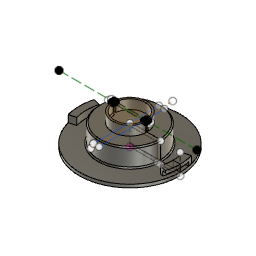
Lantern Disc (Autodesk Fusion 360 design; units mm, degrees)
Autodesk Fusion 360 part; units mm, degrees
note: some values were not read from the file. Set by a fixed rule: which sketch regions a step uses.
sketch "Profile" plane through (0, 0, 0) normal (0, 1, 0) x (1, 0, 0)
  line L0 (16.5, 0) -> (16.5, -11) construction
  line L1 (0, 0) -> (0, -11) construction
  line L2 (27, 0) -> (27, -11) construction
  line L3 (0, 0) -> (27, 0)
  line L4 (27, 0) -> (27, -1.7)
  line L5 (27, -1.7) -> (0, -1.7)
  line L6 (0, -1.7) -> (16.5, -1.7) construction
  line L7 (16.5, -1.7) -> (16.5, -11.5)
  line L8 (16.5, -11.5) -> (0, -11.5)
  line L9 (14.75, 0) -> (14.75, -9.75)
  line L10 (14.75, -9.75) -> (0, -9.75)
  line L11 (0, -11.5) -> (0, -9.75) construction
  line L12 (0, -11.5) -> (0, -9.75)
  line L13 (8.25, -16.5) -> (9.25, -16.5)
  line L14 (9.25, -16.5) -> (9.25, -11.5)
  line L15 (9.25, -11.5) -> (8.25, -11.5)
  line L16 (8.25, -11.5) -> (8.25, -16.5)
  line L17 (25, -3.7) -> (27, -3.7)
  line L18 (25, -3.7) -> (25, -1.7)
  line L19 (23.25, -5.45) -> (23.25, -1.7)
  line L20 (23.25, -5.45) -> (27, -5.45)
  line L21 (27, -5.45) -> (27, -3.7)
  line L22 (27, -3.7) -> (27, -1.7)
  dimension "d29" = 16.5
  dimension "d30" = 27
  dimension "d33" = 1.75
  dimension "d35" = 1.75
  dimension "d36" = 9.25
  dimension "d37" = 1
  dimension "d38" = 2
  dimension "d39" = 1.75
  dimension "d40" = 1.75
  dimension "d41" = 2
  dimension "d42" = 5
  dimension "d55" = 11.5
  dimension "d56" = 1.7
  constraint coincident L1.start L3.start
  constraint horizontal L3
  constraint vertical L4
  constraint horizontal L5
  constraint coincident L2 L4.end
  constraint horizontal L6
  constraint vertical L7
  constraint horizontal L8
  constraint coincident L0 L7.end
  constraint perpendicular L8 L9
  constraint coincident L1 L10.end
  constraint parallel L8 L10
  constraint perpendicular L10 L11
  constraint horizontal L13
  constraint vertical L14
  constraint horizontal L15
  constraint vertical L16
  constraint coincident L8 L14.end
  constraint coincident L2 L17.end
  constraint perpendicular L2 L17
  constraint coincident L5 L18.end
  constraint perpendicular L5 L18
  constraint coincident L5 L19.end
  constraint perpendicular L5 L19
  constraint coincident L2 L20.end
  constraint perpendicular L2 L20
  measures "d29" distance of L0 L1
  measures "d30" distance of L1 L2
  measures "d33" distance of L7 L9
  measures "d35" distance of L8 L10
  measures "d36" distance of L1 L14
  measures "d37" distance of L14 L16
  measures "d38" distance of L2 L18
  measures "d39" distance of L18 L19
  measures "d40" distance of L17 L20
  measures "d41" distance of L5 L17
  measures "d42" distance of L13.end L14.end
  measures "d55" distance of L3 L8
  measures "d56" distance of L3 L5
revolve "Body" add sketch "Profile" angle 360 about axis through (0, 0, 0) along (0, 0, 1) contours L3 L4 L5 L9 | L5 L7 L8 L9 L10 L12 L15 | L8 L13 L14 L15 L16 makes body 1
revolve "Revolve2" add sketch "Profile" angle 15 about axis through (0, 0, 0) along (0, 0, 1) second angle 15 separate body contours L5 L17 L18 L19 L20 L21 makes body 2
revolve "Revolve3" add sketch "Profile" angle 11 about axis through (0, 0, 0) along (0, 0, 1) second angle -15 separate body contours L5 L17 L18 L22 | L5 L17 L18 L19 L20 L21 makes body 3
combine "Combine1" operation add target body 3 tool bodies 2
copy_body "CopyPasteBodies3" bodies 3 makes body 4
move_body "Move2" bodies 4 to x (-1, 0, 0) y (0, -1, 0) z (0, 0, 1) at (0, 0, 0)
sketch "Sketch5" plane through (0, 0, 16.5) normal (0, 0, 1) x (-1, 0, 0)
  circle A0 centre (0, 0) radius 9.25
  circle A1 centre (0, 0) radius 8.25
  line L0 (-10.5777, -0.675) -> (10.6199, -0.675) construction
  line L1 (-11, 0.675) -> (11, 0.675) construction
  line L2 (9.2253, -0.675) -> (8.2223, -0.675)
  line L3 (9.2253, 0.675) -> (8.2223, 0.675)
  line L4 (-8.2223, 0.675) -> (-9.2253, 0.675)
  line L5 (-8.2223, -0.675) -> (-9.2253, -0.675)
  line L6 (38, 0) -> (-36, 0) construction
  point P0 (38, 0)
  point P1 (-36, 0)
  dimension "d52" = 1.35
  constraint horizontal L1
  constraint coincident L0 L2.start
  constraint coincident A0 L2.start
  constraint coincident L0 L2.end
  constraint coincident A1 L2.end
  constraint coincident L1 L3.start
  constraint coincident A0 L3.start
  constraint coincident L1 L3.end
  constraint coincident A1 L3.end
  constraint coincident L1 L4.start
  constraint coincident A1 L4.start
  constraint coincident L1 L4.end
  constraint coincident A0 L4.end
  constraint coincident L0 L5.start
  constraint coincident A1 L5.start
  constraint coincident L0 L5.end
  constraint coincident A0 L5.end
  constraint coincident P0 L6.start
  constraint coincident P1 L6.end
  measures "d52" distance of L0 L1
extrude "Extrude3" cut sketch "Sketch5" against normal blind 5 contours A0 A1 L2 L3 | A0 A1 L4 L5 bodies 1
sketch "Sketch6" plane through (0, 0, 9.75) normal (0, 0, -1) x (1, 0, 0)
  circle A0 centre (0, 0) radius 14.75
  line L0 (0, 21) -> (0, -23) construction
  line L1 (-1.5, 18) -> (-1.5, -17)
  line L2 (1.5, 18) -> (1.5, -17)
  dimension "d57" = 3
  constraint vertical L0
  constraint vertical L1
  constraint vertical L2
  constraint symmetric L0 L1 L2
  measures "d57" distance of L1 L2
extrude "Extrude4" add sketch "Sketch6" along normal blind 9.75 contours A0 L1 L2 bodies 1
chamfer "Chamfer1" distance 0.6 angle 45 10 edges at (25.1141, -6.7293, 3.7) (-25.1141, 6.7293, 3.7) (-14.75, 0, 9.75) (-1.5, 0, 9.75) (0, -8.25, 11.5) (-14.75, 0, 0) (14.75, 0, 9.75) (14.75, 0, 0) (-15.3834, -5.9667, 1.7) (-15.3834, -5.9667, 11.5) on bodies 1 3 4
equation "d29 = ( 33 / 2 ) * 1 mm"
equation "d30 = ( 54 / 2 ) * 1 mm"
equation "d36 = ( 18.5 / 2 ) * 1 mm"
named bodies: "Base", "Flange", "Flange_with_stop", "Flange_with_stop (1)"
